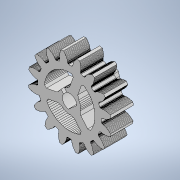
# Autodesk Inventor part: Ведущая шестерня дифференециала
Saved by Autodesk Inventor 2020 (Build 240168000, 168)
## iProperties
Created: 2021-05-23
Part Number: Ведущая шестерня дифференециала
Material: Типовые
Document SubType Name: Modeling
Designer: Антон
Density: 1 g/cm^3
Appearance: По умолчанию
Author: Антон
Autodesk Inventor part; units mm, degrees
(part 1 of 3)
ref_plane "YZ Plane" through (0, 0, 0) normal (1, 0, 0) x (0, 1, 0)
ref_plane "XZ Plane" through (0, 0, 0) normal (0, 1, 0) x (-1, 0, 0)
ref_plane "XY Plane" through (0, 0, 0) normal (0, 0, 1) x (1, 0, 0)
sketch "Эскиз1" plane through (0, 0, 0) normal (0, 0, 1) x (1, 0, 0)
  line L0 (2.5611, 6.8642) -> (2.4911, 6.9572)
  line L1 (2.4911, 6.9572) -> (2.4434, 6.9865)
  line L2 (2.4434, 6.9865) -> (2.3996, 7.0047)
  line L3 (2.3996, 7.0047) -> (2.3579, 7.0167)
  line L4 (2.3579, 7.0167) -> (2.3175, 7.0247)
  line L5 (2.3175, 7.0247) -> (2.2396, 7.0322)
  line L6 (2.2396, 7.0322) -> (2.1643, 7.0316)
  line L7 (2.1643, 7.0316) -> (2.0908, 7.025)
  line L8 (2.0908, 7.025) -> (2.0188, 7.0137)
  line L9 (2.0188, 7.0137) -> (1.8782, 6.9801)
  line L10 (1.8782, 6.9801) -> (1.7338, 6.9594)
  line L11 (1.7338, 6.9594) -> (1.5851, 6.9529)
  line L12 (1.5851, 6.9529) -> (1.4337, 6.9569)
  line L13 (1.4337, 6.9569) -> (1.28, 6.9698)
  line L14 (1.28, 6.9698) -> (1.1244, 6.9908)
  line L15 (1.1244, 6.9908) -> (0.9673, 7.0195)
  line L16 (0.9673, 7.0195) -> (0.8089, 7.0554)
  line L17 (0.8089, 7.0554) -> (0.6494, 7.0984)
  line L18 (0.6494, 7.0984) -> (0.4891, 7.1482)
  line L19 (0.4891, 7.1482) -> (0.3281, 7.2047)
  line L20 (0.3281, 7.2047) -> (0.207, 7.2514)
  line L21 (0.207, 7.2514) -> (0.1014, 7.8296)
  line L22 (0.1014, 7.8296) -> (0.1981, 7.9161)
  line L23 (0.1981, 7.9161) -> (0.3288, 8.0259)
  line L24 (0.3288, 8.0259) -> (0.4612, 8.1291)
  line L25 (0.4612, 8.1291) -> (0.5952, 8.2257)
  line L26 (0.5952, 8.2257) -> (0.7307, 8.3154)
  line L27 (0.7307, 8.3154) -> (0.8675, 8.3977)
  line L28 (0.8675, 8.3977) -> (1.0056, 8.4724)
  line L29 (1.0056, 8.4724) -> (1.1448, 8.5388)
  line L30 (1.1448, 8.5388) -> (1.2851, 8.596)
  line L31 (1.2851, 8.596) -> (1.4264, 8.6425)
  line L32 (1.4264, 8.6425) -> (1.5688, 8.6742)
  line L33 (1.5688, 8.6742) -> (1.7122, 8.6925)
  line L34 (1.7122, 8.6925) -> (1.7836, 8.7073)
  line L35 (1.7836, 8.7073) -> (1.8546, 8.7271)
  line L36 (1.8546, 8.7271) -> (1.9253, 8.7532)
  line L37 (1.9253, 8.7532) -> (1.9955, 8.7878)
  line L38 (1.9955, 8.7878) -> (2.0305, 8.8095)
  line L39 (2.0305, 8.8095) -> (2.0653, 8.8355)
  line L40 (2.0653, 8.8355) -> (2.0998, 8.868)
  line L41 (2.0998, 8.868) -> (2.1341, 8.9122)
  line L42 (2.1341, 8.9122) -> (2.1666, 9.024)
  line L43 (2.1666, 9.024) -> (2.1753, 9.5784)
  line L44 (2.1753, 9.5784) -> (2.1463, 9.6911)
  line L45 (2.1463, 9.6911) -> (2.1135, 9.7365)
  line L46 (2.1135, 9.7365) -> (2.08, 9.77)
  line L47 (2.08, 9.77) -> (2.046, 9.7971)
  line L48 (2.046, 9.7971) -> (2.0118, 9.8199)
  line L49 (2.0118, 9.8199) -> (1.9426, 9.8567)
  line L50 (1.9426, 9.8567) -> (1.8728, 9.885)
  line L51 (1.8728, 9.885) -> (1.8024, 9.907)
  line L52 (1.8024, 9.907) -> (1.7316, 9.924)
  line L53 (1.7316, 9.924) -> (1.5888, 9.9468)
  line L54 (1.5888, 9.9468) -> (1.4474, 9.983)
  line L55 (1.4474, 9.983) -> (1.3076, 10.0339)
  line L56 (1.3076, 10.0339) -> (1.1692, 10.0955)
  line L57 (1.1692, 10.0955) -> (1.0322, 10.1662)
  line L58 (1.0322, 10.1662) -> (0.8965, 10.2452)
  line L59 (0.8965, 10.2452) -> (0.7623, 10.3318)
  line L60 (0.7623, 10.3318) -> (0.6297, 10.4256)
  line L61 (0.6297, 10.4256) -> (0.4989, 10.5264)
  line L62 (0.4989, 10.5264) -> (0.3698, 10.6338)
  line L63 (0.3698, 10.6338) -> (0.2426, 10.7476)
  line L64 (0.2426, 10.7476) -> (0.1486, 10.8371)
  line L65 (0.1486, 10.8371) -> (0.2723, 11.4117)
  line L66 (0.2723, 11.4117) -> (0.3948, 11.4545)
  line L67 (0.3948, 11.4545) -> (0.5575, 11.506)
  line L68 (0.5575, 11.506) -> (0.7194, 11.5507)
  line L69 (0.7194, 11.5507) -> (0.8801, 11.5887)
  line L70 (0.8801, 11.5887) -> (1.0396, 11.6196)
  line L71 (1.0396, 11.6196) -> (1.1975, 11.6434)
  line L72 (1.1975, 11.6434) -> (1.3537, 11.6595)
  line L73 (1.3537, 11.6595) -> (1.5077, 11.6676)
  line L74 (1.5077, 11.6676) -> (1.6592, 11.6667)
  line L75 (1.6592, 11.6667) -> (1.8075, 11.6556)
  line L76 (1.8075, 11.6556) -> (1.9513, 11.6304)
  line L77 (1.9513, 11.6304) -> (2.0908, 11.5924)
  line L78 (2.0908, 11.5924) -> (2.1623, 11.5788)
  line L79 (2.1623, 11.5788) -> (2.2355, 11.5699)
  line L80 (2.2355, 11.5699) -> (2.3108, 11.567)
  line L81 (2.3108, 11.567) -> (2.389, 11.572)
  line L82 (2.389, 11.572) -> (2.4296, 11.5787)
  line L83 (2.4296, 11.5787) -> (2.4717, 11.5894)
  line L84 (2.4717, 11.5894) -> (2.516, 11.6062)
  line L85 (2.516, 11.6062) -> (2.5646, 11.634)
  line L86 (2.5646, 11.634) -> (2.6374, 11.7248)
  line L87 (2.6374, 11.7248) -> (2.8577, 12.2337)
  line L88 (2.8577, 12.2337) -> (2.874, 12.3489)
  line L89 (2.874, 12.3489) -> (2.861, 12.4034)
  line L90 (2.861, 12.4034) -> (2.8428, 12.4472)
  line L91 (2.8428, 12.4472) -> (2.8219, 12.4852)
  line L92 (2.8219, 12.4852) -> (2.799, 12.5194)
  line L93 (2.799, 12.5194) -> (2.7491, 12.5798)
  line L94 (2.7491, 12.5798) -> (2.6954, 12.6327)
  line L95 (2.6954, 12.6327) -> (2.6389, 12.6799)
  line L96 (2.6389, 12.6799) -> (2.5799, 12.7228)
  line L97 (2.5799, 12.7228) -> (2.4568, 12.7985)
  line L98 (2.4568, 12.7985) -> (2.34, 12.886)
  line L99 (2.34, 12.886) -> (2.2303, 12.9865)
  line L100 (2.2303, 12.9865) -> (2.126, 13.0964)
  line L101 (2.126, 13.0964) -> (2.0265, 13.2142)
  line L102 (2.0265, 13.2142) -> (1.9313, 13.3391)
  line L103 (1.9313, 13.3391) -> (1.8405, 13.4704)
  line L104 (1.8405, 13.4704) -> (1.7539, 13.6079)
  line L105 (1.7539, 13.6079) -> (1.6716, 13.7511)
  line L106 (1.6716, 13.7511) -> (1.5934, 13.8997)
  line L107 (1.5934, 13.8997) -> (1.5195, 14.0535)
  line L108 (1.5195, 14.0535) -> (1.4669, 14.1721)
  line L109 (1.4669, 14.1721) -> (1.8011, 14.6556)
  line L110 (1.8011, 14.6556) -> (1.9306, 14.6484)
  line L111 (1.9306, 14.6484) -> (2.1006, 14.6336)
  line L112 (2.1006, 14.6336) -> (2.2673, 14.613)
  line L113 (2.2673, 14.613) -> (2.4303, 14.5866)
  line L114 (2.4303, 14.5866) -> (2.5895, 14.5541)
  line L115 (2.5895, 14.5541) -> (2.7445, 14.5156)
  line L116 (2.7445, 14.5156) -> (2.8949, 14.4708)
  line L117 (2.8949, 14.4708) -> (3.0403, 14.4193)
  line L118 (3.0403, 14.4193) -> (3.18, 14.3605)
  line L119 (3.18, 14.3605) -> (3.3127, 14.2935)
  line L120 (3.3127, 14.2935) -> (3.4359, 14.2152)
  line L121 (3.4359, 14.2152) -> (3.5502, 14.1267)
  line L122 (3.5502, 14.1267) -> (3.6112, 14.0868)
  line L123 (3.6112, 14.0868) -> (3.6754, 14.0505)
  line L124 (3.6754, 14.0505) -> (3.7438, 14.019)
  line L125 (3.7438, 14.019) -> (3.8179, 13.9938)
  line L126 (3.8179, 13.9938) -> (3.858, 13.9844)
  line L127 (3.858, 13.9844) -> (3.901, 13.9782)
  line L128 (3.901, 13.9782) -> (3.9484, 13.9767)
  line L129 (3.9484, 13.9767) -> (4.0039, 13.9838)
  line L130 (4.0039, 13.9838) -> (4.106, 14.0398)
  line L131 (4.106, 14.0398) -> (4.5042, 14.4257)
  line L132 (4.5042, 14.4257) -> (4.5633, 14.5259)
  line L133 (4.5633, 14.5259) -> (4.5722, 14.5812)
  line L134 (4.5722, 14.5812) -> (4.5722, 14.6286)
  line L135 (4.5722, 14.6286) -> (4.5673, 14.6718)
  line L136 (4.5673, 14.6718) -> (4.5593, 14.7121)
  line L137 (4.5593, 14.7121) -> (4.5364, 14.787)
  line L138 (4.5364, 14.787) -> (4.507, 14.8564)
  line L139 (4.507, 14.8564) -> (4.4728, 14.9217)
  line L140 (4.4728, 14.9217) -> (4.4348, 14.9839)
  line L141 (4.4348, 14.9839) -> (4.3499, 15.1009)
  line L142 (4.3499, 15.1009) -> (4.2755, 15.2265)
  line L143 (4.2755, 15.2265) -> (4.2127, 15.3613)
  line L144 (4.2127, 15.3613) -> (4.1584, 15.5028)
  line L145 (4.1584, 15.5028) -> (4.1115, 15.6497)
  line L146 (4.1115, 15.6497) -> (4.0714, 15.8015)
  line L147 (4.0714, 15.8015) -> (4.0377, 15.9576)
  line L148 (4.0377, 15.9576) -> (4.0103, 16.1177)
  line L149 (4.0103, 16.1177) -> (3.989, 16.2815)
  line L150 (3.989, 16.2815) -> (3.9737, 16.4487)
  line L151 (3.9737, 16.4487) -> (3.9643, 16.6191)
  line L152 (3.9643, 16.6191) -> (3.961, 16.7488)
  line L153 (3.961, 16.7488) -> (4.4548, 17.0676)
  line L154 (4.4548, 17.0676) -> (4.5717, 17.0113)
  line L155 (4.5717, 17.0113) -> (4.7232, 16.9326)
  line L156 (4.7232, 16.9326) -> (4.8692, 16.8498)
  line L157 (4.8692, 16.8498) -> (5.0098, 16.763)
  line L158 (5.0098, 16.763) -> (5.1444, 16.6721)
  line L159 (5.1444, 16.6721) -> (5.2729, 16.5772)
  line L160 (5.2729, 16.5772) -> (5.3947, 16.4783)
  line L161 (5.3947, 16.4783) -> (5.5093, 16.375)
  line L162 (5.5093, 16.375) -> (5.6158, 16.2673)
  line L163 (5.6158, 16.2673) -> (5.7129, 16.1546)
  line L164 (5.7129, 16.1546) -> (5.7967, 16.0351)
  line L165 (5.7967, 16.0351) -> (5.8685, 15.9096)
  line L166 (5.8685, 15.9096) -> (5.9094, 15.8494)
  line L167 (5.9094, 15.8494) -> (5.9549, 15.7913)
  line L168 (5.9549, 15.7913) -> (6.0061, 15.736)
  line L169 (6.0061, 15.736) -> (6.0649, 15.6843)
  line L170 (6.0649, 15.6843) -> (6.0983, 15.6603)
  line L171 (6.0983, 15.6603) -> (6.1357, 15.6382)
  line L172 (6.1357, 15.6382) -> (6.1789, 15.6187)
  line L173 (6.1789, 15.6187) -> (6.2329, 15.604)
  line L174 (6.2329, 15.604) -> (6.3486, 15.6166)
  line L175 (6.3486, 15.6166) -> (6.8642, 15.8208)
  line L176 (6.8642, 15.8208) -> (6.9572, 15.8907)
  line L177 (6.9572, 15.8907) -> (6.9865, 15.9384)
  line L178 (6.9865, 15.9384) -> (7.0047, 15.9822)
  line L179 (7.0047, 15.9822) -> (7.0167, 16.0239)
  line L180 (7.0167, 16.0239) -> (7.0247, 16.0643)
  line L181 (7.0247, 16.0643) -> (7.0322, 16.1423)
  line L182 (7.0322, 16.1423) -> (7.0316, 16.2176)
  line L183 (7.0316, 16.2176) -> (7.025, 16.2911)
  line L184 (7.025, 16.2911) -> (7.0137, 16.363)
  line L185 (7.0137, 16.363) -> (6.9801, 16.5036)
  line L186 (6.9801, 16.5036) -> (6.9594, 16.6481)
  line L187 (6.9594, 16.6481) -> (6.9529, 16.7967)
  line L188 (6.9529, 16.7967) -> (6.9569, 16.9482)
  line L189 (6.9569, 16.9482) -> (6.9698, 17.1019)
  line L190 (6.9698, 17.1019) -> (6.9908, 17.2574)
  line L191 (6.9908, 17.2574) -> (7.0195, 17.4145)
  line L192 (7.0195, 17.4145) -> (7.0554, 17.5729)
  line L193 (7.0554, 17.5729) -> (7.0984, 17.7324)
  line L194 (7.0984, 17.7324) -> (7.1482, 17.8928)
  line L195 (7.1482, 17.8928) -> (7.2047, 18.0538)
  line L196 (7.2047, 18.0538) -> (7.2514, 18.1749)
  line L197 (7.2514, 18.1749) -> (7.8296, 18.2805)
  line L198 (7.8296, 18.2805) -> (7.9161, 18.1837)
  line L199 (7.9161, 18.1837) -> (8.0259, 18.0531)
  line L200 (8.0259, 18.0531) -> (8.1291, 17.9207)
  line L201 (8.1291, 17.9207) -> (8.2257, 17.7867)
  line L202 (8.2257, 17.7867) -> (8.3154, 17.6512)
  line L203 (8.3154, 17.6512) -> (8.3977, 17.5144)
  line L204 (8.3977, 17.5144) -> (8.4724, 17.3763)
  line L205 (8.4724, 17.3763) -> (8.5388, 17.2371)
  line L206 (8.5388, 17.2371) -> (8.596, 17.0968)
  line L207 (8.596, 17.0968) -> (8.6425, 16.9555)
  line L208 (8.6425, 16.9555) -> (8.6742, 16.813)
  line L209 (8.6742, 16.813) -> (8.6925, 16.6696)
  line L210 (8.6925, 16.6696) -> (8.7073, 16.5983)
  line L211 (8.7073, 16.5983) -> (8.7271, 16.5273)
  line L212 (8.7271, 16.5273) -> (8.7532, 16.4566)
  line L213 (8.7532, 16.4566) -> (8.7878, 16.3863)
  line L214 (8.7878, 16.3863) -> (8.8095, 16.3514)
  line L215 (8.8095, 16.3514) -> (8.8355, 16.3166)
  line L216 (8.8355, 16.3166) -> (8.868, 16.282)
  line L217 (8.868, 16.282) -> (8.9122, 16.2478)
  line L218 (8.9122, 16.2478) -> (9.024, 16.2152)
  line L219 (9.024, 16.2152) -> (9.5784, 16.2065)
  line L220 (9.5784, 16.2065) -> (9.6911, 16.2356)
  line L221 (9.6911, 16.2356) -> (9.7365, 16.2684)
  line L222 (9.7365, 16.2684) -> (9.77, 16.3019)
  line L223 (9.77, 16.3019) -> (9.7971, 16.3359)
  line L224 (9.7971, 16.3359) -> (9.8199, 16.3701)
  line L225 (9.8199, 16.3701) -> (9.8567, 16.4393)
  line L226 (9.8567, 16.4393) -> (9.885, 16.5091)
  line L227 (9.885, 16.5091) -> (9.907, 16.5795)
  line L228 (9.907, 16.5795) -> (9.924, 16.6503)
  line L229 (9.924, 16.6503) -> (9.9468, 16.7931)
  line L230 (9.9468, 16.7931) -> (9.983, 16.9344)
  line L231 (9.983, 16.9344) -> (10.0339, 17.0742)
  line L232 (10.0339, 17.0742) -> (10.0955, 17.2126)
  line L233 (10.0955, 17.2126) -> (10.1662, 17.3497)
  line L234 (10.1662, 17.3497) -> (10.2452, 17.4854)
  line L235 (10.2452, 17.4854) -> (10.3318, 17.6195)
  line L236 (10.3318, 17.6195) -> (10.4256, 17.7521)
  line L237 (10.4256, 17.7521) -> (10.5264, 17.883)
  line L238 (10.5264, 17.883) -> (10.6338, 18.0121)
  line L239 (10.6338, 18.0121) -> (10.7476, 18.1392)
  line L240 (10.7476, 18.1392) -> (10.8371, 18.2332)
  line L241 (10.8371, 18.2332) -> (11.4117, 18.1095)
  line L242 (11.4117, 18.1095) -> (11.4545, 17.987)
  line L243 (11.4545, 17.987) -> (11.506, 17.8243)
  line L244 (11.506, 17.8243) -> (11.5507, 17.6625)
  line L245 (11.5507, 17.6625) -> (11.5887, 17.5017)
  line L246 (11.5887, 17.5017) -> (11.6196, 17.3423)
  line L247 (11.6196, 17.3423) -> (11.6434, 17.1843)
  line L248 (11.6434, 17.1843) -> (11.6595, 17.0282)
  line L249 (11.6595, 17.0282) -> (11.6676, 16.8742)
  line L250 (11.6676, 16.8742) -> (11.6667, 16.7227)
  line L251 (11.6667, 16.7227) -> (11.6556, 16.5743)
  line L252 (11.6556, 16.5743) -> (11.6304, 16.4306)
  line L253 (11.6304, 16.4306) -> (11.5924, 16.2911)
  line L254 (11.5924, 16.2911) -> (11.5788, 16.2195)
  line L255 (11.5788, 16.2195) -> (11.5699, 16.1463)
  line L256 (11.5699, 16.1463) -> (11.567, 16.071)
  line L257 (11.567, 16.071) -> (11.572, 15.9929)
  line L258 (11.572, 15.9929) -> (11.5787, 15.9523)
  line L259 (11.5787, 15.9523) -> (11.5894, 15.9102)
  line L260 (11.5894, 15.9102) -> (11.6062, 15.8658)
  line L261 (11.6062, 15.8658) -> (11.634, 15.8173)
  line L262 (11.634, 15.8173) -> (11.7248, 15.7444)
  line L263 (11.7248, 15.7444) -> (12.2337, 15.5242)
  line L264 (12.2337, 15.5242) -> (12.3489, 15.5079)
  line L265 (12.3489, 15.5079) -> (12.4034, 15.5209)
  line L266 (12.4034, 15.5209) -> (12.4472, 15.539)
  line L267 (12.4472, 15.539) -> (12.4852, 15.56)
  line L268 (12.4852, 15.56) -> (12.5194, 15.5829)
  line L269 (12.5194, 15.5829) -> (12.5798, 15.6327)
  line L270 (12.5798, 15.6327) -> (12.6327, 15.6864)
  line L271 (12.6327, 15.6864) -> (12.6799, 15.743)
  line L272 (12.6799, 15.743) -> (12.7228, 15.8019)
  line L273 (12.7228, 15.8019) -> (12.7985, 15.9251)
  line L274 (12.7985, 15.9251) -> (12.886, 16.0419)
  line L275 (12.886, 16.0419) -> (12.9865, 16.1515)
  line L276 (12.9865, 16.1515) -> (13.0964, 16.2558)
  line L277 (13.0964, 16.2558) -> (13.2142, 16.3554)
  line L278 (13.2142, 16.3554) -> (13.3391, 16.4505)
  line L279 (13.3391, 16.4505) -> (13.4704, 16.5413)
  line L280 (13.4704, 16.5413) -> (13.6079, 16.6279)
  line L281 (13.6079, 16.6279) -> (13.7511, 16.7103)
  line L282 (13.7511, 16.7103) -> (13.8997, 16.7885)
  line L283 (13.8997, 16.7885) -> (14.0535, 16.8624)
  line L284 (14.0535, 16.8624) -> (14.1721, 16.915)
  line L285 (14.1721, 16.915) -> (14.6556, 16.5808)
  line L286 (14.6556, 16.5808) -> (14.6484, 16.4512)
  line L287 (14.6484, 16.4512) -> (14.6336, 16.2812)
  line L288 (14.6336, 16.2812) -> (14.613, 16.1146)
  line L289 (14.613, 16.1146) -> (14.5866, 15.9515)
  line L290 (14.5866, 15.9515) -> (14.5541, 15.7924)
  line L291 (14.5541, 15.7924) -> (14.5156, 15.6374)
  line L292 (14.5156, 15.6374) -> (14.4708, 15.4869)
  line L293 (14.4708, 15.4869) -> (14.4193, 15.3416)
  line L294 (14.4193, 15.3416) -> (14.3605, 15.2019)
  line L295 (14.3605, 15.2019) -> (14.2935, 15.0691)
  line L296 (14.2935, 15.0691) -> (14.2152, 14.946)
  line L297 (14.2152, 14.946) -> (14.1267, 14.8316)
  line L298 (14.1267, 14.8316) -> (14.0868, 14.7707)
  line L299 (14.0868, 14.7707) -> (14.0505, 14.7065)
  line L300 (14.0505, 14.7065) -> (14.019, 14.638)
  line L301 (14.019, 14.638) -> (13.9938, 14.5639)
  line L302 (13.9938, 14.5639) -> (13.9844, 14.5238)
  line L303 (13.9844, 14.5238) -> (13.9782, 14.4809)
  line L304 (13.9782, 14.4809) -> (13.9767, 14.4335)
  line L305 (13.9767, 14.4335) -> (13.9838, 14.378)
  line L306 (13.9838, 14.378) -> (14.0398, 14.2759)
  line L307 (14.0398, 14.2759) -> (14.4257, 13.8777)
  line L308 (14.4257, 13.8777) -> (14.5259, 13.8185)
  line L309 (14.5259, 13.8185) -> (14.5812, 13.8097)
  line L310 (14.5812, 13.8097) -> (14.6286, 13.8097)
  line L311 (14.6286, 13.8097) -> (14.6718, 13.8145)
  line L312 (14.6718, 13.8145) -> (14.7121, 13.8226)
  line L313 (14.7121, 13.8226) -> (14.787, 13.8455)
  line L314 (14.787, 13.8455) -> (14.8564, 13.8749)
  line L315 (14.8564, 13.8749) -> (14.9217, 13.9091)
  line L316 (14.9217, 13.9091) -> (14.9839, 13.9471)
  line L317 (14.9839, 13.9471) -> (15.1009, 14.032)
  line L318 (15.1009, 14.032) -> (15.2265, 14.1063)
  line L319 (15.2265, 14.1063) -> (15.3613, 14.1692)
  line L320 (15.3613, 14.1692) -> (15.5028, 14.2235)
  line L321 (15.5028, 14.2235) -> (15.6497, 14.2704)
  line L322 (15.6497, 14.2704) -> (15.8015, 14.3105)
  line L323 (15.8015, 14.3105) -> (15.9576, 14.3441)
  line L324 (15.9576, 14.3441) -> (16.1177, 14.3715)
  line L325 (16.1177, 14.3715) -> (16.2815, 14.3928)
  line L326 (16.2815, 14.3928) -> (16.4487, 14.4082)
  line L327 (16.4487, 14.4082) -> (16.6191, 14.4176)
  line L328 (16.6191, 14.4176) -> (16.7488, 14.4208)
  line L329 (16.7488, 14.4208) -> (17.0676, 13.927)
  line L330 (17.0676, 13.927) -> (17.0113, 13.8101)
  line L331 (17.0113, 13.8101) -> (16.9326, 13.6587)
  line L332 (16.9326, 13.6587) -> (16.8498, 13.5126)
  line L333 (16.8498, 13.5126) -> (16.763, 13.3721)
  line L334 (16.763, 13.3721) -> (16.6721, 13.2375)
  line L335 (16.6721, 13.2375) -> (16.5772, 13.109)
  line L336 (16.5772, 13.109) -> (16.4783, 12.9872)
  line L337 (16.4783, 12.9872) -> (16.375, 12.8726)
  line L338 (16.375, 12.8726) -> (16.2673, 12.766)
  line L339 (16.2673, 12.766) -> (16.1546, 12.669)
  line L340 (16.1546, 12.669) -> (16.0351, 12.5852)
  line L341 (16.0351, 12.5852) -> (15.9096, 12.5134)
  line L342 (15.9096, 12.5134) -> (15.8494, 12.4724)
  line L343 (15.8494, 12.4724) -> (15.7913, 12.4269)
  line L344 (15.7913, 12.4269) -> (15.736, 12.3758)
  line L345 (15.736, 12.3758) -> (15.6843, 12.317)
  line L346 (15.6843, 12.317) -> (15.6603, 12.2835)
  line L347 (15.6603, 12.2835) -> (15.6382, 12.2462)
  line L348 (15.6382, 12.2462) -> (15.6187, 12.203)
  line L349 (15.6187, 12.203) -> (15.604, 12.149)
  line L350 (15.604, 12.149) -> (15.6166, 12.0333)
  line L351 (15.6166, 12.0333) -> (15.8208, 11.5177)
  line L352 (15.8208, 11.5177) -> (15.8907, 11.4247)
  line L353 (15.8907, 11.4247) -> (15.9384, 11.3953)
  line L354 (15.9384, 11.3953) -> (15.9822, 11.3772)
  line L355 (15.9822, 11.3772) -> (16.0239, 11.3651)
  line L356 (16.0239, 11.3651) -> (16.0643, 11.3572)
  line L357 (16.0643, 11.3572) -> (16.1423, 11.3497)
  line L358 (16.1423, 11.3497) -> (16.2176, 11.3503)
  line L359 (16.2176, 11.3503) -> (16.2911, 11.3568)
  line L360 (16.2911, 11.3568) -> (16.363, 11.3682)
  line L361 (16.363, 11.3682) -> (16.5036, 11.4018)
  line L362 (16.5036, 11.4018) -> (16.6481, 11.4224)
  line L363 (16.6481, 11.4224) -> (16.7967, 11.4289)
  line L364 (16.7967, 11.4289) -> (16.9482, 11.425)
  line L365 (16.9482, 11.425) -> (17.1019, 11.4121)
  line L366 (17.1019, 11.4121) -> (17.2574, 11.3911)
  line L367 (17.2574, 11.3911) -> (17.4145, 11.3624)
  line L368 (17.4145, 11.3624) -> (17.5729, 11.3264)
  line L369 (17.5729, 11.3264) -> (17.7324, 11.2834)
  line L370 (17.7324, 11.2834) -> (17.8928, 11.2336)
  line L371 (17.8928, 11.2336) -> (18.0538, 11.1771)
  line L372 (18.0538, 11.1771) -> (18.1749, 11.1304)
  line L373 (18.1749, 11.1304) -> (18.2805, 10.5522)
  line L374 (18.2805, 10.5522) -> (18.1837, 10.4658)
  line L375 (18.1837, 10.4658) -> (18.0531, 10.356)
  line L376 (18.0531, 10.356) -> (17.9207, 10.2527)
  line L377 (17.9207, 10.2527) -> (17.7867, 10.1561)
  line L378 (17.7867, 10.1561) -> (17.6512, 10.0665)
  line L379 (17.6512, 10.0665) -> (17.5144, 9.9841)
  line L380 (17.5144, 9.9841) -> (17.3763, 9.9095)
  line L381 (17.3763, 9.9095) -> (17.2371, 9.8431)
  line L382 (17.2371, 9.8431) -> (17.0968, 9.7859)
  line L383 (17.0968, 9.7859) -> (16.9555, 9.7394)
  line L384 (16.9555, 9.7394) -> (16.813, 9.7076)
  line L385 (16.813, 9.7076) -> (16.6696, 9.6894)
  line L386 (16.6696, 9.6894) -> (16.5983, 9.6746)
  line L387 (16.5983, 9.6746) -> (16.5273, 9.6547)
  line L388 (16.5273, 9.6547) -> (16.4566, 9.6287)
  line L389 (16.4566, 9.6287) -> (16.3863, 9.5941)
  line L390 (16.3863, 9.5941) -> (16.3514, 9.5724)
  line L391 (16.3514, 9.5724) -> (16.3166, 9.5464)
  line L392 (16.3166, 9.5464) -> (16.282, 9.5139)
  line L393 (16.282, 9.5139) -> (16.2478, 9.4696)
  line L394 (16.2478, 9.4696) -> (16.2152, 9.3579)
  line L395 (16.2152, 9.3579) -> (16.2065, 8.8034)
  line L396 (16.2065, 8.8034) -> (16.2356, 8.6907)
  line L397 (16.2356, 8.6907) -> (16.2684, 8.6454)
  line L398 (16.2684, 8.6454) -> (16.3019, 8.6119)
  line L399 (16.3019, 8.6119) -> (16.3359, 8.5848)
  line L400 (16.3359, 8.5848) -> (16.3701, 8.5619)
  line L401 (16.3701, 8.5619) -> (16.4393, 8.5252)
  line L402 (16.4393, 8.5252) -> (16.5091, 8.4969)
  line L403 (16.5091, 8.4969) -> (16.5795, 8.4749)
  line L404 (16.5795, 8.4749) -> (16.6503, 8.4578)
  line L405 (16.6503, 8.4578) -> (16.7931, 8.4351)
  line L406 (16.7931, 8.4351) -> (16.9344, 8.3988)
  line L407 (16.9344, 8.3988) -> (17.0742, 8.348)
  line L408 (17.0742, 8.348) -> (17.2126, 8.2864)
  line L409 (17.2126, 8.2864) -> (17.3497, 8.2156)
  line L410 (17.3497, 8.2156) -> (17.4854, 8.1367)
  line L411 (17.4854, 8.1367) -> (17.6195, 8.0501)
  line L412 (17.6195, 8.0501) -> (17.7521, 7.9562)
  line L413 (17.7521, 7.9562) -> (17.883, 7.8555)
  line L414 (17.883, 7.8555) -> (18.0121, 7.7481)
  line L415 (18.0121, 7.7481) -> (18.1392, 7.6343)
  line L416 (18.1392, 7.6343) -> (18.2332, 7.5448)
  line L417 (18.2332, 7.5448) -> (18.1095, 6.9702)
  line L418 (18.1095, 6.9702) -> (17.987, 6.9273)
  line L419 (17.987, 6.9273) -> (17.8243, 6.8759)
  line L420 (17.8243, 6.8759) -> (17.6625, 6.8312)
  line L421 (17.6625, 6.8312) -> (17.5017, 6.7932)
  line L422 (17.5017, 6.7932) -> (17.3423, 6.7622)
  line L423 (17.3423, 6.7622) -> (17.1843, 6.7385)
  line L424 (17.1843, 6.7385) -> (17.0282, 6.7224)
  line L425 (17.0282, 6.7224) -> (16.8742, 6.7143)
  line L426 (16.8742, 6.7143) -> (16.7227, 6.7151)
  line L427 (16.7227, 6.7151) -> (16.5743, 6.7263)
  line L428 (16.5743, 6.7263) -> (16.4306, 6.7515)
  line L429 (16.4306, 6.7515) -> (16.2911, 6.7895)
  line L430 (16.2911, 6.7895) -> (16.2195, 6.8031)
  line L431 (16.2195, 6.8031) -> (16.1463, 6.812)
  line L432 (16.1463, 6.812) -> (16.071, 6.8149)
  line L433 (16.071, 6.8149) -> (15.9929, 6.8099)
  line L434 (15.9929, 6.8099) -> (15.9523, 6.8032)
  line L435 (15.9523, 6.8032) -> (15.9102, 6.7924)
  line L436 (15.9102, 6.7924) -> (15.8658, 6.7757)
  line L437 (15.8658, 6.7757) -> (15.8173, 6.7479)
  line L438 (15.8173, 6.7479) -> (15.7444, 6.6571)
  line L439 (15.7444, 6.6571) -> (15.5242, 6.1482)
  line L440 (15.5242, 6.1482) -> (15.5079, 6.0329)
  line L441 (15.5079, 6.0329) -> (15.5209, 5.9785)
  line L442 (15.5209, 5.9785) -> (15.539, 5.9347)
  line L443 (15.539, 5.9347) -> (15.56, 5.8967)
  line L444 (15.56, 5.8967) -> (15.5829, 5.8625)
  line L445 (15.5829, 5.8625) -> (15.6327, 5.8021)
  line L446 (15.6327, 5.8021) -> (15.6864, 5.7492)
  line L447 (15.6864, 5.7492) -> (15.743, 5.7019)
  line L448 (15.743, 5.7019) -> (15.8019, 5.6591)
  line L449 (15.8019, 5.6591) -> (15.9251, 5.5834)
  line L450 (15.9251, 5.5834) -> (16.0419, 5.4958)
  line L451 (16.0419, 5.4958) -> (16.1515, 5.3953)
  line L452 (16.1515, 5.3953) -> (16.2558, 5.2855)
  line L453 (16.2558, 5.2855) -> (16.3554, 5.1677)
  line L454 (16.3554, 5.1677) -> (16.4505, 5.0428)
  line L455 (16.4505, 5.0428) -> (16.5413, 4.9114)
  line L456 (16.5413, 4.9114) -> (16.6279, 4.774)
  line L457 (16.6279, 4.774) -> (16.7103, 4.6308)
  line L458 (16.7103, 4.6308) -> (16.7885, 4.4822)
  line L459 (16.7885, 4.4822) -> (16.8624, 4.3284)
  line L460 (16.8624, 4.3284) -> (16.915, 4.2097)
  line L461 (16.915, 4.2097) -> (16.5808, 3.7262)
  line L462 (16.5808, 3.7262) -> (16.4512, 3.7335)
  line L463 (16.4512, 3.7335) -> (16.2812, 3.7483)
  line L464 (16.2812, 3.7483) -> (16.1146, 3.7689)
  line L465 (16.1146, 3.7689) -> (15.9515, 3.7953)
  line L466 (15.9515, 3.7953) -> (15.7924, 3.8277)
  line L467 (15.7924, 3.8277) -> (15.6374, 3.8662)
  line L468 (15.6374, 3.8662) -> (15.4869, 3.9111)
  line L469 (15.4869, 3.9111) -> (15.3416, 3.9626)
  line L470 (15.3416, 3.9626) -> (15.2019, 4.0213)
  line L471 (15.2019, 4.0213) -> (15.0691, 4.0884)
  line L472 (15.0691, 4.0884) -> (14.946, 4.1667)
  line L473 (14.946, 4.1667) -> (14.8316, 4.2551)
  line L474 (14.8316, 4.2551) -> (14.7707, 4.2951)
  line L475 (14.7707, 4.2951) -> (14.7065, 4.3313)
  line L476 (14.7065, 4.3313) -> (14.638, 4.3629)
  line L477 (14.638, 4.3629) -> (14.5639, 4.3881)
  line L478 (14.5639, 4.3881) -> (14.5238, 4.3975)
  line L479 (14.5238, 4.3975) -> (14.4809, 4.4036)
  line L480 (14.4809, 4.4036) -> (14.4335, 4.4051)
  line L481 (14.4335, 4.4051) -> (14.378, 4.398)
  line L482 (14.378, 4.398) -> (14.2759, 4.3421)
  line L483 (14.2759, 4.3421) -> (13.8777, 3.9562)
  line L484 (13.8777, 3.9562) -> (13.8185, 3.8559)
  line L485 (13.8185, 3.8559) -> (13.8097, 3.8007)
  line L486 (13.8097, 3.8007) -> (13.8097, 3.7533)
  line L487 (13.8097, 3.7533) -> (13.8145, 3.7101)
  line L488 (13.8145, 3.7101) -> (13.8226, 3.6697)
  line L489 (13.8226, 3.6697) -> (13.8455, 3.5949)
  line L490 (13.8455, 3.5949) -> (13.8749, 3.5255)
  line L491 (13.8749, 3.5255) -> (13.9091, 3.4601)
  line L492 (13.9091, 3.4601) -> (13.9471, 3.398)
  line L493 (13.9471, 3.398) -> (14.032, 3.2809)
  line L494 (14.032, 3.2809) -> (14.1063, 3.1554)
  line L495 (14.1063, 3.1554) -> (14.1692, 3.0205)
  line L496 (14.1692, 3.0205) -> (14.2235, 2.8791)
  line L497 (14.2235, 2.8791) -> (14.2704, 2.7322)
  line L498 (14.2704, 2.7322) -> (14.3105, 2.5804)
  line L499 (14.3105, 2.5804) -> (14.3441, 2.4243)
  line L500 (14.3441, 2.4243) -> (14.3715, 2.2642)
  line L501 (14.3715, 2.2642) -> (14.3928, 2.1004)
  line L502 (14.3928, 2.1004) -> (14.4082, 1.9332)
  line L503 (14.4082, 1.9332) -> (14.4176, 1.7628)
  line L504 (14.4176, 1.7628) -> (14.4208, 1.6331)
  line L505 (14.4208, 1.6331) -> (13.927, 1.3142)
  line L506 (13.927, 1.3142) -> (13.8101, 1.3705)
  line L507 (13.8101, 1.3705) -> (13.6587, 1.4492)
  line L508 (13.6587, 1.4492) -> (13.5126, 1.532)
  line L509 (13.5126, 1.532) -> (13.3721, 1.6189)
  line L510 (13.3721, 1.6189) -> (13.2375, 1.7097)
  line L511 (13.2375, 1.7097) -> (13.109, 1.8046)
  line L512 (13.109, 1.8046) -> (12.9872, 1.9036)
  line L513 (12.9872, 1.9036) -> (12.8726, 2.0068)
  line L514 (12.8726, 2.0068) -> (12.766, 2.1145)
  line L515 (12.766, 2.1145) -> (12.669, 2.2273)
  line L516 (12.669, 2.2273) -> (12.5852, 2.3468)
  line L517 (12.5852, 2.3468) -> (12.5134, 2.4723)
  line L518 (12.5134, 2.4723) -> (12.4724, 2.5325)
  line L519 (12.4724, 2.5325) -> (12.4269, 2.5905)
  line L520 (12.4269, 2.5905) -> (12.3758, 2.6459)
  line L521 (12.3758, 2.6459) -> (12.317, 2.6976)
  line L522 (12.317, 2.6976) -> (12.2835, 2.7215)
  line L523 (12.2835, 2.7215) -> (12.2462, 2.7437)
  line L524 (12.2462, 2.7437) -> (12.203, 2.7632)
  line L525 (12.203, 2.7632) -> (12.149, 2.7779)
  line L526 (12.149, 2.7779) -> (12.0333, 2.7652)
  line L527 (12.0333, 2.7652) -> (11.5177, 2.5611)
  line L528 (11.5177, 2.5611) -> (11.4247, 2.4911)
  line L529 (11.4247, 2.4911) -> (11.3953, 2.4434)
  line L530 (11.3953, 2.4434) -> (11.3772, 2.3996)
  line L531 (11.3772, 2.3996) -> (11.3651, 2.3579)
  line L532 (11.3651, 2.3579) -> (11.3572, 2.3175)
  line L533 (11.3572, 2.3175) -> (11.3497, 2.2396)
  line L534 (11.3497, 2.2396) -> (11.3503, 2.1643)
  line L535 (11.3503, 2.1643) -> (11.3568, 2.0908)
  line L536 (11.3568, 2.0908) -> (11.3682, 2.0188)
  line L537 (11.3682, 2.0188) -> (11.4018, 1.8782)
  line L538 (11.4018, 1.8782) -> (11.4224, 1.7338)
  line L539 (11.4224, 1.7338) -> (11.4289, 1.5851)
  line L540 (11.4289, 1.5851) -> (11.425, 1.4337)
  line L541 (11.425, 1.4337) -> (11.4121, 1.28)
  line L542 (11.4121, 1.28) -> (11.3911, 1.1244)
  line L543 (11.3911, 1.1244) -> (11.3624, 0.9673)
  line L544 (11.3624, 0.9673) -> (11.3264, 0.8089)
  line L545 (11.3264, 0.8089) -> (11.2834, 0.6494)
  line L546 (11.2834, 0.6494) -> (11.2336, 0.4891)
  line L547 (11.2336, 0.4891) -> (11.1771, 0.3281)
  line L548 (11.1771, 0.3281) -> (11.1304, 0.207)
  line L549 (11.1304, 0.207) -> (10.5522, 0.1014)
  line L550 (10.5522, 0.1014) -> (10.4658, 0.1981)
  line L551 (10.4658, 0.1981) -> (10.356, 0.3288)
  line L552 (10.356, 0.3288) -> (10.2527, 0.4612)
  line L553 (10.2527, 0.4612) -> (10.1561, 0.5952)
  line L554 (10.1561, 0.5952) -> (10.0665, 0.7307)
  line L555 (10.0665, 0.7307) -> (9.9841, 0.8675)
  line L556 (9.9841, 0.8675) -> (9.9095, 1.0056)
  line L557 (9.9095, 1.0056) -> (9.8431, 1.1448)
  line L558 (9.8431, 1.1448) -> (9.7859, 1.2851)
  line L559 (9.7859, 1.2851) -> (9.7394, 1.4264)
  line L560 (9.7394, 1.4264) -> (9.7076, 1.5688)
  line L561 (9.7076, 1.5688) -> (9.6894, 1.7122)
  line L562 (9.6894, 1.7122) -> (9.6746, 1.7836)
  line L563 (9.6746, 1.7836) -> (9.6547, 1.8546)
  line L564 (9.6547, 1.8546) -> (9.6287, 1.9253)
  line L565 (9.6287, 1.9253) -> (9.5941, 1.9955)
  line L566 (9.5941, 1.9955) -> (9.5724, 2.0305)
  line L567 (9.5724, 2.0305) -> (9.5464, 2.0653)
  line L568 (9.5464, 2.0653) -> (9.5139, 2.0998)
  line L569 (9.5139, 2.0998) -> (9.4696, 2.1341)
  line L570 (9.4696, 2.1341) -> (9.3579, 2.1666)
  line L571 (9.3579, 2.1666) -> (8.8034, 2.1753)
  line L572 (8.8034, 2.1753) -> (8.6907, 2.1463)
  line L573 (8.6907, 2.1463) -> (8.6454, 2.1135)
  line L574 (8.6454, 2.1135) -> (8.6119, 2.08)
  line L575 (8.6119, 2.08) -> (8.5848, 2.046)
  line L576 (8.5848, 2.046) -> (8.5619, 2.0118)
  line L577 (8.5619, 2.0118) -> (8.5252, 1.9426)
  line L578 (8.5252, 1.9426) -> (8.4969, 1.8728)
  line L579 (8.4969, 1.8728) -> (8.4749, 1.8024)
  line L580 (8.4749, 1.8024) -> (8.4578, 1.7316)
  line L581 (8.4578, 1.7316) -> (8.4351, 1.5888)
  line L582 (8.4351, 1.5888) -> (8.3988, 1.4474)
  line L583 (8.3988, 1.4474) -> (8.348, 1.3076)
  line L584 (8.348, 1.3076) -> (8.2864, 1.1692)
  line L585 (8.2864, 1.1692) -> (8.2156, 1.0322)
  line L586 (8.2156, 1.0322) -> (8.1367, 0.8965)
  line L587 (8.1367, 0.8965) -> (8.0501, 0.7623)
  line L588 (8.0501, 0.7623) -> (7.9562, 0.6297)
  line L589 (7.9562, 0.6297) -> (7.8555, 0.4989)
  line L590 (7.8555, 0.4989) -> (7.7481, 0.3698)
  line L591 (7.7481, 0.3698) -> (7.6343, 0.2426)
  line L592 (7.6343, 0.2426) -> (7.5448, 0.1486)
  line L593 (7.5448, 0.1486) -> (6.9702, 0.2723)
  line L594 (6.9702, 0.2723) -> (6.9273, 0.3948)
  line L595 (6.9273, 0.3948) -> (6.8759, 0.5575)
  line L596 (6.8759, 0.5575) -> (6.8312, 0.7194)
  line L597 (6.8312, 0.7194) -> (6.7932, 0.8801)
  line L598 (6.7932, 0.8801) -> (6.7622, 1.0396)
  line L599 (6.7622, 1.0396) -> (6.7385, 1.1975)
  line L600 (6.7385, 1.1975) -> (6.7224, 1.3537)
  line L601 (6.7224, 1.3537) -> (6.7143, 1.5077)
  line L602 (6.7143, 1.5077) -> (6.7151, 1.6592)
  line L603 (6.7151, 1.6592) -> (6.7263, 1.8075)
  line L604 (6.7263, 1.8075) -> (6.7515, 1.9513)
  line L605 (6.7515, 1.9513) -> (6.7895, 2.0908)
  line L606 (6.7895, 2.0908) -> (6.8031, 2.1623)
  line L607 (6.8031, 2.1623) -> (6.812, 2.2355)
  line L608 (6.812, 2.2355) -> (6.8149, 2.3108)
  line L609 (6.8149, 2.3108) -> (6.8099, 2.389)
  line L610 (6.8099, 2.389) -> (6.8032, 2.4296)
  line L611 (6.8032, 2.4296) -> (6.7924, 2.4717)
  line L612 (6.7924, 2.4717) -> (6.7757, 2.516)
  line L613 (6.7757, 2.516) -> (6.7479, 2.5646)
  line L614 (6.7479, 2.5646) -> (6.6571, 2.6374)
  line L615 (6.6571, 2.6374) -> (6.1482, 2.8577)
  line L616 (6.1482, 2.8577) -> (6.0329, 2.874)
  line L617 (6.0329, 2.874) -> (5.9785, 2.861)
  line L618 (5.9785, 2.861) -> (5.9347, 2.8428)
  line L619 (5.9347, 2.8428) -> (5.8967, 2.8219)
  line L620 (5.8967, 2.8219) -> (5.8625, 2.799)
  line L621 (5.8625, 2.799) -> (5.8021, 2.7491)
  line L622 (5.8021, 2.7491) -> (5.7492, 2.6954)
  line L623 (5.7492, 2.6954) -> (5.7019, 2.6389)
  line L624 (5.7019, 2.6389) -> (5.6591, 2.5799)
  line L625 (5.6591, 2.5799) -> (5.5834, 2.4568)
  line L626 (5.5834, 2.4568) -> (5.4958, 2.34)
  line L627 (5.4958, 2.34) -> (5.3953, 2.2303)
  line L628 (5.3953, 2.2303) -> (5.2855, 2.126)
  line L629 (5.2855, 2.126) -> (5.1677, 2.0265)
  line L630 (5.1677, 2.0265) -> (5.0428, 1.9313)
  line L631 (5.0428, 1.9313) -> (4.9114, 1.8405)
  line L632 (4.9114, 1.8405) -> (4.774, 1.7539)
  line L633 (4.774, 1.7539) -> (4.6308, 1.6716)
  line L634 (4.6308, 1.6716) -> (4.4822, 1.5934)
  line L635 (4.4822, 1.5934) -> (4.3284, 1.5195)
  line L636 (4.3284, 1.5195) -> (4.2097, 1.4669)
  line L637 (4.2097, 1.4669) -> (3.7262, 1.8011)
  line L638 (3.7262, 1.8011) -> (3.7335, 1.9306)
  line L639 (3.7335, 1.9306) -> (3.7483, 2.1006)
  line L640 (3.7483, 2.1006) -> (3.7689, 2.2673)
  line L641 (3.7689, 2.2673) -> (3.7953, 2.4303)
  line L642 (3.7953, 2.4303) -> (3.8277, 2.5895)
  line L643 (3.8277, 2.5895) -> (3.8662, 2.7445)
  line L644 (3.8662, 2.7445) -> (3.9111, 2.8949)
  line L645 (3.9111, 2.8949) -> (3.9626, 3.0403)
  line L646 (3.9626, 3.0403) -> (4.0213, 3.18)
  line L647 (4.0213, 3.18) -> (4.0884, 3.3127)
  line L648 (4.0884, 3.3127) -> (4.1667, 3.4359)
  line L649 (4.1667, 3.4359) -> (4.2551, 3.5502)
  line L650 (4.2551, 3.5502) -> (4.2951, 3.6112)
  line L651 (4.2951, 3.6112) -> (4.3313, 3.6754)
  line L652 (4.3313, 3.6754) -> (4.3629, 3.7438)
  line L653 (4.3629, 3.7438) -> (4.3881, 3.8179)
  line L654 (4.3881, 3.8179) -> (4.3975, 3.858)
  line L655 (4.3975, 3.858) -> (4.4036, 3.901)
  line L656 (4.4036, 3.901) -> (4.4051, 3.9484)
  line L657 (4.4051, 3.9484) -> (4.398, 4.0039)
  line L658 (4.398, 4.0039) -> (4.3421, 4.106)
  line L659 (4.3421, 4.106) -> (3.9562, 4.5042)
  line L660 (3.9562, 4.5042) -> (3.8559, 4.5633)
  line L661 (3.8559, 4.5633) -> (3.8007, 4.5722)
  line L662 (3.8007, 4.5722) -> (3.7533, 4.5722)
  line L663 (3.7533, 4.5722) -> (3.7101, 4.5673)
  line L664 (3.7101, 4.5673) -> (3.6697, 4.5593)
  line L665 (3.6697, 4.5593) -> (3.5949, 4.5364)
  line L666 (3.5949, 4.5364) -> (3.5255, 4.507)
  line L667 (3.5255, 4.507) -> (3.4601, 4.4728)
  line L668 (3.4601, 4.4728) -> (3.398, 4.4348)
  line L669 (3.398, 4.4348) -> (3.2809, 4.3499)
  line L670 (3.2809, 4.3499) -> (3.1554, 4.2755)
  line L671 (3.1554, 4.2755) -> (3.0205, 4.2127)
  line L672 (3.0205, 4.2127) -> (2.8791, 4.1584)
  line L673 (2.8791, 4.1584) -> (2.7322, 4.1115)
  line L674 (2.7322, 4.1115) -> (2.5804, 4.0714)
  line L675 (2.5804, 4.0714) -> (2.4243, 4.0377)
  line L676 (2.4243, 4.0377) -> (2.2642, 4.0103)
  line L677 (2.2642, 4.0103) -> (2.1004, 3.989)
  line L678 (2.1004, 3.989) -> (1.9332, 3.9737)
  line L679 (1.9332, 3.9737) -> (1.7628, 3.9643)
  line L680 (1.7628, 3.9643) -> (1.6331, 3.961)
  line L681 (1.6331, 3.961) -> (1.3142, 4.4548)
  line L682 (1.3142, 4.4548) -> (1.3705, 4.5717)
  line L683 (1.3705, 4.5717) -> (1.4492, 4.7232)
  line L684 (1.4492, 4.7232) -> (1.532, 4.8692)
  line L685 (1.532, 4.8692) -> (1.6189, 5.0098)
  line L686 (1.6189, 5.0098) -> (1.7097, 5.1444)
  line L687 (1.7097, 5.1444) -> (1.8046, 5.2729)
  line L688 (1.8046, 5.2729) -> (1.9036, 5.3947)
  line L689 (1.9036, 5.3947) -> (2.0068, 5.5093)
  line L690 (2.0068, 5.5093) -> (2.1145, 5.6158)
  line L691 (2.1145, 5.6158) -> (2.2273, 5.7129)
  line L692 (2.2273, 5.7129) -> (2.3468, 5.7967)
  line L693 (2.3468, 5.7967) -> (2.4723, 5.8685)
  line L694 (2.4723, 5.8685) -> (2.5325, 5.9094)
  line L695 (2.5325, 5.9094) -> (2.5905, 5.9549)
  line L696 (2.5905, 5.9549) -> (2.6459, 6.0061)
  line L697 (2.6459, 6.0061) -> (2.6976, 6.0649)
  line L698 (2.6976, 6.0649) -> (2.7215, 6.0983)
  line L699 (2.7215, 6.0983) -> (2.7437, 6.1357)
  line L700 (2.7437, 6.1357) -> (2.7632, 6.1789)
  line L701 (2.7632, 6.1789) -> (2.7779, 6.2329)
  line L702 (2.7779, 6.2329) -> (2.7652, 6.3486)
  line L703 (2.7652, 6.3486) -> (2.5611, 6.8642)
  line L704 (6.7155, 7.7678) -> (4.4109, 7.3469)
  line L705 (4.4109, 7.3469) -> (4.1296, 6.81)
  line L706 (4.1296, 6.81) -> (4.2968, 6.4829)
  line L707 (4.2968, 6.4829) -> (4.4851, 6.1676)
  line L708 (4.4851, 6.1676) -> (4.6936, 5.8652)
  line L709 (4.6936, 5.8652) -> (4.9216, 5.5772)
  line L710 (4.9216, 5.5772) -> (5.168, 5.3048)
  line L711 (5.168, 5.3048) -> (5.4317, 5.0492)
  line L712 (5.4317, 5.0492) -> (5.7116, 4.8114)
  line L713 (5.7116, 4.8114) -> (6.0066, 4.5925)
  line L714 (6.0066, 4.5925) -> (6.3152, 4.3934)
  line L715 (6.3152, 4.3934) -> (6.6363, 4.215)
  line L716 (6.6363, 4.215) -> (6.9684, 4.0581)
  line L717 (6.9684, 4.0581) -> (7.31, 3.9233)
  line L718 (7.31, 3.9233) -> (7.6598, 3.8112)
  line L719 (7.6598, 3.8112) -> (8.0162, 3.7223)
  line L720 (8.0162, 3.7223) -> (8.3776, 3.657)
  line L721 (8.3776, 3.657) -> (8.7426, 3.6156)
  line L722 (8.7426, 3.6156) -> (9.1094, 3.5981)
  line L723 (9.1094, 3.5981) -> (9.4767, 3.6049)
  line L724 (9.4767, 3.6049) -> (9.8427, 3.6357)
  line L725 (9.8427, 3.6357) -> (10.2059, 3.6904)
  line L726 (10.2059, 3.6904) -> (10.5647, 3.7689)
  line L727 (10.5647, 3.7689) -> (10.9176, 3.8707)
  line L728 (10.9176, 3.8707) -> (11.263, 3.9955)
  line L729 (11.263, 3.9955) -> (11.5995, 4.1427)
  line L730 (11.5995, 4.1427) -> (11.7219, 4.7363)
  line L731 (11.7219, 4.7363) -> (10.2051, 6.5218)
  line L732 (10.2051, 6.5218) -> (9.3539, 6.7859)
  line L733 (9.3539, 6.7859) -> (9.0243, 6.7862)
  line L734 (9.0243, 6.7862) -> (8.6977, 6.8314)
  line L735 (8.6977, 6.8314) -> (8.3803, 6.9208)
  line L736 (8.3803, 6.9208) -> (8.0781, 7.0526)
  line L737 (8.0781, 7.0526) -> (7.7968, 7.2245)
  line L738 (7.7968, 7.2245) -> (7.5415, 7.4331)
  line L739 (7.5415, 7.4331) -> (6.7155, 7.7678)
  line L740 (11.6611, 7.7587) -> (13.178, 5.9733)
  line L741 (13.178, 5.9733) -> (13.7836, 5.9982)
  line L742 (13.7836, 5.9982) -> (13.9832, 6.3065)
  line L743 (13.9832, 6.3065) -> (14.1622, 6.6272)
  line L744 (14.1622, 6.6272) -> (14.3197, 6.959)
  line L745 (14.3197, 6.959) -> (14.4551, 7.3004)
  line L746 (14.4551, 7.3004) -> (14.5679, 7.65)
  line L747 (14.5679, 7.65) -> (14.6574, 8.0062)
  line L748 (14.6574, 8.0062) -> (14.7234, 8.3675)
  line L749 (14.7234, 8.3675) -> (14.7655, 8.7324)
  line L750 (14.7655, 8.7324) -> (14.7836, 9.0993)
  line L751 (14.7836, 9.0993) -> (14.7775, 9.4665)
  line L752 (14.7775, 9.4665) -> (14.7474, 9.8325)
  line L753 (14.7474, 9.8325) -> (14.6933, 10.1958)
  line L754 (14.6933, 10.1958) -> (14.6155, 10.5548)
  line L755 (14.6155, 10.5548) -> (14.5143, 10.9079)
  line L756 (14.5143, 10.9079) -> (14.3901, 11.2535)
  line L757 (14.3901, 11.2535) -> (14.2435, 11.5903)
  line L758 (14.2435, 11.5903) -> (14.0752, 11.9168)
  line L759 (14.0752, 11.9168) -> (13.8857, 12.2314)
  line L760 (13.8857, 12.2314) -> (13.6761, 12.533)
  line L761 (13.6761, 12.533) -> (13.4471, 12.8202)
  line L762 (13.4471, 12.8202) -> (13.1997, 13.0917)
  line L763 (13.1997, 13.0917) -> (12.9351, 13.3463)
  line L764 (12.9351, 13.3463) -> (12.6543, 13.5831)
  line L765 (12.6543, 13.5831) -> (12.3585, 13.8009)
  line L766 (12.3585, 13.8009) -> (11.7832, 13.6101)
  line L767 (11.7832, 13.6101) -> (10.9954, 11.4038)
  line L768 (10.9954, 11.4038) -> (11.1922, 10.5346)
  line L769 (11.1922, 10.5346) -> (11.3569, 10.249)
  line L770 (11.3569, 10.249) -> (11.481, 9.9435)
  line L771 (11.481, 9.9435) -> (11.5623, 9.624)
  line L772 (11.5623, 9.624) -> (11.5992, 9.2964)
  line L773 (11.5992, 9.2964) -> (11.591, 8.9668)
  line L774 (11.591, 8.9668) -> (11.538, 8.6414)
  line L775 (11.538, 8.6414) -> (11.6611, 7.7587)
  line L776 (9.1961, 12.0463) -> (9.9839, 14.2526)
  line L777 (9.9839, 14.2526) -> (9.6596, 14.7646)
  line L778 (9.6596, 14.7646) -> (9.2928, 14.7834)
  line L779 (9.2928, 14.7834) -> (8.9255, 14.778)
  line L780 (8.9255, 14.778) -> (8.5594, 14.7485)
  line L781 (8.5594, 14.7485) -> (8.196, 14.6951)
  line L782 (8.196, 14.6951) -> (7.837, 14.618)
  line L783 (7.837, 14.618) -> (7.4837, 14.5174)
  line L784 (7.4837, 14.5174) -> (7.1378, 14.3939)
  line L785 (7.1378, 14.3939) -> (6.8007, 14.2479)
  line L786 (6.8007, 14.2479) -> (6.474, 14.0801)
  line L787 (6.474, 14.0801) -> (6.159, 13.8913)
  line L788 (6.159, 13.8913) -> (5.857, 13.6822)
  line L789 (5.857, 13.6822) -> (5.5695, 13.4537)
  line L790 (5.5695, 13.4537) -> (5.2975, 13.2068)
  line L791 (5.2975, 13.2068) -> (5.0423, 12.9426)
  line L792 (5.0423, 12.9426) -> (4.8051, 12.6623)
  line L793 (4.8051, 12.6623) -> (4.5867, 12.3669)
  line L794 (4.5867, 12.3669) -> (4.3882, 12.0579)
  line L795 (4.3882, 12.0579) -> (4.2104, 11.7365)
  line L796 (4.2104, 11.7365) -> (4.0541, 11.4041)
  line L797 (4.0541, 11.4041) -> (3.9199, 11.0622)
  line L798 (3.9199, 11.0622) -> (3.8084, 10.7123)
  line L799 (3.8084, 10.7123) -> (3.7202, 10.3557)
  line L800 (3.7202, 10.3557) -> (3.6555, 9.9942)
  line L801 (3.6555, 9.9942) -> (3.6147, 9.6291)
  line L802 (3.6147, 9.6291) -> (4.0677, 9.2263)
  line L803 (4.0677, 9.2263) -> (6.3723, 9.6472)
  line L804 (6.3723, 9.6472) -> (7.0266, 10.2523)
  line L805 (7.0266, 10.2523) -> (7.1917, 10.5377)
  line L806 (7.1917, 10.5377) -> (7.3941, 10.7979)
  line L807 (7.3941, 10.7979) -> (7.6302, 11.028)
  line L808 (7.6302, 11.028) -> (7.8955, 11.2238)
  line L809 (7.8955, 11.2238) -> (8.185, 11.3816)
  line L810 (8.185, 11.3816) -> (8.4933, 11.4983)
  line L811 (8.4933, 11.4983) -> (9.1961, 12.0463)
  circle A0 centre (9.1909, 9.1909) radius 0.5
  line L812 (6.1273, 9.1909) -> (12.2546, 9.1909)
  line L813 (9.1909, 6.1273) -> (9.1909, 12.2546)
  constraints: 1628 end point, 1 centre point
extrude "Выдавливание1" add sketch "Эскиз1" along normal blind 5